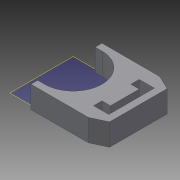
# Autodesk Inventor part: giunto_fondo_siringa
Saved by Autodesk Inventor 2014 SP1 (Build 180222100, 222)
## iProperties
Created: 2015-04-15
Part Number: giunto_fondo_siringa
Material: Generic
Document SubType Name: Modeling
Designer: Giorgio Nuzzo
Density: 1 g/cm^3
Appearance: Default
Author: Giorgio Nuzzo
Autodesk Inventor part; units mm, degrees
ref_plane "YZ Plane" through (0, 0, 0) normal (1, 0, 0) x (0, 1, 0)
ref_plane "XZ Plane" through (0, 0, 0) normal (0, 1, 0) x (-1, 0, 0)
ref_plane "XY Plane" through (0, 0, 0) normal (0, 0, 1) x (1, 0, 0)
ref_plane "Work Plane1" through (-4.5, 4.3393, 236.083) normal (0, 0, -1) x (1, 0, 0)
sketch "Sketch1" plane through (-4.5, 4.3393, 236.083) normal (0, 0, -1) x (1, 0, 0)
  circle A0 centre (0, 4.1863) radius 17 construction
  line L0 (34.5, -9.3137) -> (34.5, 17.6863) projected
  line L1 (34.5, 17.6863) -> (25.5, 17.6863) projected
  line L2 (25.5, 17.6863) -> (25.5, 12.6863) projected
  line L3 (25.5, 12.6863) -> (30.5, 12.6863) projected
  line L4 (30.5, 12.6863) -> (30.5, -4.3137) projected
  line L5 (30.5, -4.3137) -> (25.5, -4.3137) projected
  line L6 (25.5, -4.3137) -> (25.5, -9.3137) projected
  line L7 (25.5, -9.3137) -> (34.5, -9.3137) projected
  line L8 (0, -8.3452) -> (0, -17.0863) construction
  line L9 (0, -12.8137) -> (-4, -12.8137)
  line L10 (-4, -12.8137) -> (-4, -16.8137)
  line L11 (-4, -16.8137) -> (30, -16.8137)
  line L12 (30, -16.8137) -> (38.5, -12.8501)
  line L13 (38.5, -12.8501) -> (38.5, 4.1863)
  arc A1 (0, -12.8137) -> (17, 4.1863) centre (0, 4.1863) ccw
  line L14 (0, 4.1863) -> (38.5, 4.1863) construction
  line L15 (0, 21.1863) -> (-4, 21.1863)
  line L16 (-4, 21.1863) -> (-4, 25.1863)
  line L17 (-4, 25.1863) -> (30, 25.1863)
  line L18 (30, 25.1863) -> (38.5, 21.2227)
  line L19 (38.5, 21.2227) -> (38.5, 4.1863)
  arc A2 (17, 4.1863) -> (0, 21.1863) centre (0, 4.1863) ccw
  point P0 (4.5, 4.3393)
  point P1 (0, 25.4589)
  dimension "d0" = 4
  dimension "d1" = 4
  dimension "d2" = 4
  dimension "d3" = 115
  dimension "d4" = 8.5
  constraints: 24 end point, 6 point on circle, 6 symmetric about line, 5 perpendicular, 2 centre point, 2 tangent, 1 concentric, 1 parallel, 1 point on line, 1 other
  measures "d0" distance of L9.start L9.end
  measures "d1" distance of L9.end L10.end
  measures "d2" distance between parallel lines of L0 L13
  measures "d3" angle of L12 L13
  measures "d4" horizontal distance of L11.end L12.end
extrude "Extrusion1" add sketch "Sketch1" against normal blind 13
body "Solid1"
